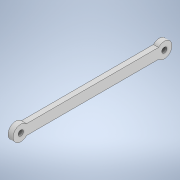
# Autodesk Inventor part: DERKS Linkage Arm
Saved by Autodesk Inventor 2020 (Build 240168000, 168)
## iProperties
Created: 2020-04-30
Part Number: DERKS Linkage Arm
Material: Generic
Document SubType Name: Modeling
Designer: tader
Density: 1 g/cm^3
Appearance: Default
Author: tader
Autodesk Inventor part; units mm, degrees
ref_plane "YZ Plane" through (0, 0, 0) normal (1, 0, 0) x (0, 1, 0)
ref_plane "XZ Plane" through (0, 0, 0) normal (0, 1, 0) x (-1, 0, 0)
ref_plane "XY Plane" through (0, 0, 0) normal (0, 0, 1) x (1, 0, 0)
sketch "Sketch1" plane through (0, 0, 0) normal (1, 0, 0) x (0, 1, 0)
  line L0 (-0.0183, 6.6801) -> (-0.0183, -34.2201)
  line L1 (-0.0183, -34.2201) -> (6.3317, -34.2201)
  line L2 (6.3317, -34.2201) -> (6.3317, 6.6801)
  arc A0 (6.3317, 6.6801) -> (-0.0183, 6.6801) centre (3.1567, 10.2299) ccw
  point P0 (0, 0)
  dimension "d0" = 6.35
  constraints: 6 end point, 2 point on circle, 1 centre point, 1 parallel
  measures "d0" distance of L1.end L0.end
extrude "Extrusion1" add sketch "Sketch1" along normal blind 3.175
sketch "Sketch2" plane through (3.175, 0, 0) normal (1, 0, 0) x (0, 0, -1)
  arc A0 (-6.6801, 6.3317) -> (-6.6801, -0.0183) centre (-10.2299, 3.1567) ccw projected
  line L0 (-6.6801, -0.0183) -> (34.2201, -0.0183) projected
  line L1 (34.2201, -0.0183) -> (34.2201, 6.3317) projected
  line L2 (34.2201, 6.3317) -> (-6.6801, 6.3317) projected
  point P0 (0, 0)
  constraints: 1 coincident
hole "Hole1" at (3.175, 3.1567, 10.2299) direction (-1, 0, 0) diameter 3.2512 end through all
mirror "Mirror1" about plane through (0, -0.0183, -34.2201) normal (0, 0, -1) of "Extrusion1", "Hole1"
body "Solid1"
